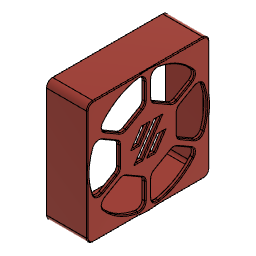
[a]_60mm_fan_blank_insert_x2 (Autodesk Fusion 360 design; units mm, degrees)
Autodesk Fusion 360 part; units mm, degrees
note: some values were not read from the file. Set by a fixed rule: which sketch regions a step uses.
sketch "Master" plane through (0, 0, 0) normal (1, 0, 0) x (0, 1, 0) in component "[a]_60mm_fan_blank_insert_x2"
  line L0 (30, -30) -> (-30, -30)
  line L1 (-30, -30) -> (-30, 30)
  line L2 (-30, 30) -> (30, 30)
  line L3 (30, 30) -> (30, -30)
  line L4 (30, -30) -> (-30, 30) construction
  line L5 (-30, -30) -> (30, 30) construction
  line L6 (-3, 14.4679) -> (-11.0296, 9.8321)
  line L7 (-14.0296, 4.6359) -> (-14.0296, -4.6359)
  line L8 (-11.0296, -9.8321) -> (-3, -14.4679)
  line L9 (3, -14.4679) -> (11.0296, -9.8321)
  line L10 (14.0296, -4.6359) -> (14.0296, 4.6359)
  line L11 (11.0296, 9.8321) -> (3, 14.4679)
  line L12 (-1.5, 25.3537) -> (-1.5, 17.066)
  line L13 (0, 0) -> (0, 50) construction
  line L14 (1.5, 25.3537) -> (1.5, 17.066)
  line L15 (-22.707, 11.3778) -> (-15.5296, 7.234)
  line L16 (-21.207, 13.9759) -> (-14.0296, 9.8321)
  line L17 (-21.207, -13.9759) -> (-14.0296, -9.8321)
  line L18 (-22.707, -11.3778) -> (-15.5296, -7.234)
  line L19 (1.5, -25.3537) -> (1.5, -17.066)
  line L20 (-1.5, -25.3537) -> (-1.5, -17.066)
  line L21 (22.707, -11.3778) -> (15.5296, -7.234)
  line L22 (21.207, -13.9759) -> (14.0296, -9.8321)
  line L23 (21.207, 13.9759) -> (14.0296, 9.8321)
  line L24 (22.707, 11.3778) -> (15.5296, 7.234)
  line L25 (-3.3031, 7.0506) -> (0.0865, 7.0506)
  line L26 (0.0865, 7.0506) -> (-4.5489, -0.001)
  line L27 (-4.5489, -0.001) -> (-7.9375, -0.001)
  line L28 (-7.9375, -0.001) -> (-3.3031, 7.0506)
  line L29 (2.9411, 7.0506) -> (6.3297, 7.0506)
  line L30 (6.3297, 7.0506) -> (-2.9401, -7.0506)
  line L31 (-2.9401, -7.0506) -> (-6.3287, -7.0506)
  line L32 (-6.3287, -7.0506) -> (2.9411, 7.0506)
  line L33 (4.5489, -0.001) -> (7.9375, -0.001)
  line L34 (7.9375, -0.001) -> (3.3031, -7.0506)
  line L35 (3.3031, -7.0506) -> (-0.0855, -7.0506)
  line L36 (-0.0855, -7.0506) -> (4.5489, -0.001)
  arc A0 (22.0029, 18.5049) -> (5.0243, 28.3076) centre (0, 0) ccw
  arc A1 (27.0272, -9.8026) -> (27.0272, 9.8026) centre (0, 0) ccw
  arc A2 (5.0243, -28.3076) -> (22.0029, -18.5049) centre (0, 0) ccw
  arc A3 (-22.0029, -18.5049) -> (-5.0243, -28.3076) centre (0, 0) ccw
  arc A4 (-5.0243, 28.3076) -> (-22.0029, 18.5049) centre (0, 0) ccw
  arc A5 (-27.0272, 9.8026) -> (-27.0272, -9.8026) centre (0, 0) ccw
  arc A6 (21.207, 13.9759) -> (22.0029, 18.5049) centre (19.707, 16.574) ccw
  arc A7 (5.0243, 28.3076) -> (1.5, 25.3537) centre (4.5, 25.3537) ccw
  arc A8 (1.5, 17.066) -> (3, 14.4679) centre (4.5, 17.066) ccw
  arc A9 (11.0296, 9.8321) -> (14.0296, 9.8321) centre (12.5296, 12.4301) ccw
  arc A10 (-1.5, 25.3537) -> (-5.0243, 28.3076) centre (-4.5, 25.3537) ccw
  arc A11 (-3, 14.4679) -> (-1.5, 17.066) centre (-4.5, 17.066) ccw
  arc A12 (-14.0296, 9.8321) -> (-11.0296, 9.8321) centre (-12.5296, 12.4301) ccw
  arc A13 (-22.0029, 18.5049) -> (-21.207, 13.9759) centre (-19.707, 16.574) ccw
  arc A14 (-14.0296, 4.6359) -> (-15.5296, 7.234) centre (-17.0296, 4.6359) ccw
  arc A15 (-22.707, 11.3778) -> (-27.0272, 9.8026) centre (-24.207, 8.7798) ccw
  arc A16 (-27.0272, -9.8026) -> (-22.707, -11.3778) centre (-24.207, -8.7798) ccw
  arc A17 (-15.5296, -7.234) -> (-14.0296, -4.6359) centre (-17.0296, -4.6359) ccw
  arc A18 (-11.0296, -9.8321) -> (-14.0296, -9.8321) centre (-12.5296, -12.4301) ccw
  arc A19 (-21.207, -13.9759) -> (-22.0029, -18.5049) centre (-19.707, -16.574) ccw
  arc A20 (-5.0243, -28.3076) -> (-1.5, -25.3537) centre (-4.5, -25.3537) ccw
  arc A21 (-1.5, -17.066) -> (-3, -14.4679) centre (-4.5, -17.066) ccw
  arc A22 (3, -14.4679) -> (1.5, -17.066) centre (4.5, -17.066) ccw
  arc A23 (14.0296, -9.8321) -> (11.0296, -9.8321) centre (12.5296, -12.4301) ccw
  arc A24 (22.0029, -18.5049) -> (21.207, -13.9759) centre (19.707, -16.574) ccw
  arc A25 (1.5, -25.3537) -> (5.0243, -28.3076) centre (4.5, -25.3537) ccw
  arc A26 (22.707, -11.3778) -> (27.0272, -9.8026) centre (24.207, -8.7798) ccw
  arc A27 (27.0272, 9.8026) -> (22.707, 11.3778) centre (24.207, 8.7798) ccw
  arc A28 (15.5296, 7.234) -> (14.0296, 4.6359) centre (17.0296, 4.6359) ccw
  arc A29 (14.0296, -4.6359) -> (15.5296, -7.234) centre (17.0296, -4.6359) ccw
  dimension "d2" = 60
  dimension "d3" = 60
  dimension "d4" = 57.5
  dimension "d14" = 1.5
  dimension "d15" = 3
  constraint horizontal L0
  constraint perpendicular L0 L1
  constraint parallel L0 L2
  constraint parallel L1 L3
  constraint coincident L4 L13.start
  constraint coincident L5 L13.start
  constraint coincident L13.start A0.centre
  constraint vertical L13
  constraint vertical L12
  constraint concentric A0 A4
  constraint concentric A1 A4
  constraint concentric A2 A4
  constraint concentric A3 A4
  constraint concentric A4 A5
  constraint tangent L23 A6
  constraint tangent A0 A6
  constraint tangent A0 A7
  constraint tangent L14 A7
  constraint equal A6 A7
  constraint tangent L11 A8
  constraint tangent L14 A8
  constraint equal A6 A8
  constraint tangent L23 A9
  constraint tangent L11 A9
  constraint equal A6 A9
  constraint tangent L12 A10
  constraint tangent A4 A10
  constraint equal A6 A10
  constraint tangent L12 A11
  constraint tangent L6 A11
  constraint equal A6 A11
  constraint tangent L6 A12
  constraint tangent L16 A12
  constraint equal A6 A12
  constraint tangent L16 A13
  constraint tangent A4 A13
  constraint equal A6 A13
  constraint tangent L15 A14
  constraint tangent L7 A14
  constraint equal A6 A14
  constraint tangent L15 A15
  constraint tangent A5 A15
  constraint equal A6 A15
  constraint tangent L18 A16
  constraint tangent A5 A16
  constraint equal A6 A16
  constraint tangent L18 A17
  constraint tangent L7 A17
  constraint equal A6 A17
  constraint tangent L17 A18
  constraint tangent L8 A18
  constraint equal A6 A18
  constraint tangent L17 A19
  constraint tangent A3 A19
  constraint equal A6 A19
  constraint tangent L20 A20
  constraint tangent A3 A20
  constraint equal A6 A20
  constraint tangent L20 A21
  constraint tangent L8 A21
  constraint equal A6 A21
  constraint tangent L19 A22
  constraint tangent L9 A22
  constraint equal A6 A22
  constraint tangent L22 A23
  constraint tangent L9 A23
  constraint equal A6 A23
  constraint tangent L22 A24
  constraint tangent A2 A24
  constraint equal A6 A24
  constraint tangent L19 A25
  constraint tangent A2 A25
  constraint equal A6 A25
  constraint tangent L21 A26
  constraint tangent A1 A26
  constraint equal A6 A26
  constraint tangent L24 A27
  constraint tangent A1 A27
  constraint equal A6 A27
  constraint tangent L24 A28
  constraint tangent L10 A28
  constraint equal A6 A28
  constraint tangent L21 A29
  constraint tangent L10 A29
  constraint equal A6 A29
  measures "d2" distance of L1.end L2.end
  measures "d3" distance of L0.end L1.end
  measures "d4" diameter of A4
  measures "d14" distance of L13 L14
  measures "d15" radius of A6
sketch "Outer Square" plane through (0, 0, 0) normal (1, 0, 0) x (0, 1, 0) in component "[a]_60mm_fan_blank_insert_x2"
  line L0 (-30, 30) -> (30, 30)
  line L1 (-30, -30) -> (-30, 30)
  line L2 (30, -30) -> (-30, -30)
  line L3 (30, 30) -> (30, -30)
extrude "Extrude1" add sketch "Outer Square" against normal blind 20 in component "[a]_60mm_fan_blank_insert_x2"
fillet "Fillet1" radius 3 4 edges at (-10, 30, 30) (-10, -30, 30) (-10, 30, -30) (-10, -30, -30) in component "[a]_60mm_fan_blank_insert_x2"
shell "Shell1" thickness 1.6 removed faces 1 at (-20, -11, -10) in component "[a]_60mm_fan_blank_insert_x2"
extrude "Extrude2" cut sketch "Master" against normal blind 1.6 contours L6 L12 L16 A4 A10 A11 A12 A13 | L7 L15 L18 A5 A14 A15 A16 A17 | L8 L17 L20 A3 A18 A19 A20 A21 | L9 L19 L22 A2 A22 A23 A24 A25 | L10 L21 L24 A1 A26 A27 A28 A29 | L11 L14 L23 A0 A6 A7 A8 A9 | L25 L26 L27 L28 | L29 L30 L31 L32 | L33 L34 L35 L36 in component "[a]_60mm_fan_blank_insert_x2"
chamfer "Chamfer1" distance 0.4 angle 45 68 edges at (0, -14.375, 24.8982) (0, -2.5729, 27.653) (0, -1.5, 21.2099) (0, -1.9019, 15.566) (0, -7.0148, 12.15) (0, -12.5296, 9.4301) (0, -17.6183, 11.904) (0, -22.6617, 16.0547) (0, -25.2346, 11.5983) (0, -19.1183, 9.3059) (0, -14.4315, 6.1359) (0, -14.0296, 0) (0, -14.4315, -6.1359) (0, -19.1183, -9.3059) (0, -25.2346, -11.5983) (0, -28.75, 0) (0, -17.6183, -11.904) (0, -12.5296, -9.4301) (0, -7.0148, -12.15) (0, -1.9019, -15.566) (0, -1.5, -21.2099) (0, -2.5729, -27.653) (0, -14.375, -24.8982) (0, -22.6617, -16.0547) (0, 1.5, -21.2099) (0, 1.9019, -15.566) (0, 7.0148, -12.15) (0, 12.5296, -9.4301) (0, 17.6183, -11.904) (0, 22.6617, -16.0547) (0, 14.375, -24.8982) (0, 2.5729, -27.653) (0, 19.1183, -9.3059) (0, 14.4315, -6.1359) (0, 14.0296, 0) (0, 14.4315, 6.1359) (0, 19.1183, 9.3059) (0, 25.2346, 11.5983) (0, 28.75, 0) (0, 25.2346, -11.5983) (0, 12.5296, 9.4301) (0, 7.0148, 12.15) (0, 1.9019, 15.566) (0, 1.5, 21.2099) (0, 2.5729, 27.653) (0, 14.375, 24.8982) (0, 22.6617, 16.0547) (0, 17.6183, 11.904) (0, 30, 0) (0, 29.1213, -29.1213) (0, 0, -30) (0, -29.1213, -29.1213) (0, -30, 0) (0, -29.1213, 29.1213) (0, 0, 30) (0, 29.1213, 29.1213) (0, -5.6203, 3.5248) (0, -6.2432, -0.001) (0, -2.2312, 3.5248) (0, -1.6083, 7.0506) (0, -1.6938, 0) (0, -4.6344, -7.0506) (0, 1.6948, 0) (0, 4.6354, 7.0506) (0, 2.2317, -3.5258) (0, 6.2432, -0.001) (0, 5.6203, -3.5258) (0, 1.6088, -7.0506) in component "[a]_60mm_fan_blank_insert_x2"
sketch "Sketch3" plane through (0, 0, 0) normal (1, 0, 0) x (0, 1, 0) in component "[a]_60mm_fan_blank_insert_x2"
  line L0 (7.0713, 7.4506) -> (-2.7244, -7.4506)
  line L1 (-2.7244, -7.4506) -> (-7.0703, -7.4506)
  line L2 (-7.0703, -7.4506) -> (2.7254, 7.4506)
  line L3 (2.7254, 7.4506) -> (7.0713, 7.4506)
  arc A0 (29.6, 27) -> (27, 29.6) centre (27, 27) ccw
  arc A1 (-27, 29.6) -> (-29.6, 27) centre (-27, 27) ccw
  arc A2 (-29.6, -27) -> (-27, -29.6) centre (-27, -27) ccw
  arc A3 (27, -29.6) -> (29.6, -27) centre (27, -27) ccw
  line L4 (22.507, -11.7242) -> (15.3296, -7.5804)
  arc A4 (13.6296, -4.6359) -> (15.3296, -7.5804) centre (17.0296, -4.6359) ccw
  line L5 (13.6296, -4.6359) -> (13.6296, 4.6359)
  arc A5 (15.3296, 7.5804) -> (13.6296, 4.6359) centre (17.0296, 4.6359) ccw
  line L6 (15.3296, 7.5804) -> (22.507, 11.7242)
  arc A6 (27.4033, 9.939) -> (22.507, 11.7242) centre (24.207, 8.7798) ccw
  arc A7 (27.4033, -9.939) -> (27.4033, 9.939) centre (0, 0) ccw
  arc A8 (22.507, -11.7242) -> (27.4033, -9.939) centre (24.207, -8.7798) ccw
  line L7 (-21.407, -13.6295) -> (-14.2296, -9.4856)
  arc A9 (-10.8296, -9.4856) -> (-14.2296, -9.4856) centre (-12.5296, -12.4301) ccw
  line L8 (-10.8296, -9.4856) -> (-2.8, -14.1215)
  arc A10 (-1.1, -17.066) -> (-2.8, -14.1215) centre (-4.5, -17.066) ccw
  line L9 (-1.1, -17.066) -> (-1.1, -25.3537)
  arc A11 (-5.0942, -28.7014) -> (-1.1, -25.3537) centre (-4.5, -25.3537) ccw
  arc A12 (-22.3091, -18.7624) -> (-5.0942, -28.7014) centre (0, 0) ccw
  arc A13 (-21.407, -13.6295) -> (-22.3091, -18.7624) centre (-19.707, -16.574) ccw
  arc A14 (-5.0942, 28.7014) -> (-22.3091, 18.7624) centre (0, 0) ccw
  arc A15 (-1.1, 25.3537) -> (-5.0942, 28.7014) centre (-4.5, 25.3537) ccw
  line L10 (-1.1, 25.3537) -> (-1.1, 17.066)
  arc A16 (-2.8, 14.1215) -> (-1.1, 17.066) centre (-4.5, 17.066) ccw
  line L11 (-2.8, 14.1215) -> (-10.8296, 9.4856)
  arc A17 (-14.2296, 9.4856) -> (-10.8296, 9.4856) centre (-12.5296, 12.4301) ccw
  line L12 (-14.2296, 9.4856) -> (-21.407, 13.6295)
  arc A18 (-22.3091, 18.7624) -> (-21.407, 13.6295) centre (-19.707, 16.574) ccw
  arc A19 (-22.507, 11.7242) -> (-27.4033, 9.939) centre (-24.207, 8.7798) ccw
  line L13 (-22.507, 11.7242) -> (-15.3296, 7.5804)
  arc A20 (-13.6296, 4.6359) -> (-15.3296, 7.5804) centre (-17.0296, 4.6359) ccw
  line L14 (-13.6296, 4.6359) -> (-13.6296, -4.6359)
  arc A21 (-15.3296, -7.5804) -> (-13.6296, -4.6359) centre (-17.0296, -4.6359) ccw
  line L15 (-15.3296, -7.5804) -> (-22.507, -11.7242)
  arc A22 (-27.4033, -9.939) -> (-22.507, -11.7242) centre (-24.207, -8.7798) ccw
  arc A23 (-27.4033, 9.939) -> (-27.4033, -9.939) centre (0, 0) ccw
  line L16 (1.1, -25.3537) -> (1.1, -17.066)
  arc A24 (2.8, -14.1215) -> (1.1, -17.066) centre (4.5, -17.066) ccw
  line L17 (2.8, -14.1215) -> (10.8296, -9.4856)
  arc A25 (14.2296, -9.4856) -> (10.8296, -9.4856) centre (12.5296, -12.4301) ccw
  line L18 (14.2296, -9.4856) -> (21.407, -13.6295)
  arc A26 (22.3091, -18.7624) -> (21.407, -13.6295) centre (19.707, -16.574) ccw
  arc A27 (5.0942, -28.7014) -> (22.3091, -18.7624) centre (0, 0) ccw
  arc A28 (1.1, -25.3537) -> (5.0942, -28.7014) centre (4.5, -25.3537) ccw
  arc A29 (10.8296, 9.4856) -> (14.2296, 9.4856) centre (12.5296, 12.4301) ccw
  line L19 (10.8296, 9.4856) -> (2.8, 14.1215)
  arc A30 (1.1, 17.066) -> (2.8, 14.1215) centre (4.5, 17.066) ccw
  line L20 (1.1, 17.066) -> (1.1, 25.3537)
  arc A31 (5.0942, 28.7014) -> (1.1, 25.3537) centre (4.5, 25.3537) ccw
  arc A32 (22.3091, 18.7624) -> (5.0942, 28.7014) centre (0, 0) ccw
  arc A33 (21.407, 13.6295) -> (22.3091, 18.7624) centre (19.707, 16.574) ccw
  line L21 (21.407, 13.6295) -> (14.2296, 9.4856)
  line L22 (0.8281, 7.4506) -> (-4.3332, -0.401)
  line L23 (-4.3332, -0.401) -> (-8.679, -0.401)
  line L24 (-8.679, -0.401) -> (-3.5189, 7.4506)
  line L25 (-3.5189, 7.4506) -> (0.8281, 7.4506)
  line L26 (8.6792, 0.399) -> (3.5188, -7.4506)
  line L27 (3.5188, -7.4506) -> (-0.8271, -7.4506)
  line L28 (-0.8271, -7.4506) -> (4.3332, 0.399)
  line L29 (4.3332, 0.399) -> (8.6792, 0.399)
  circle A34 centre (0, 0) radius 30
  circle A35 centre (0, 0) radius 29.2
  dimension "d19" = 60
  dimension "d20" = 58.4
  constraint coincident A7.centre A12.centre
  constraint concentric A7 A35
  measures "d19" diameter of A34
  measures "d20" diameter of A35
extrude "Extrude3" add sketch "Sketch3" against normal blind 1.6 contours A34 in component "[a]_60mm_fan_blank_insert_x2"
component "[a]_60mm_fan_blank_insert_x2" placed x (1, 0, 0) y (0, 1, 0) z (0, 0, 1) at (0, 0, 0)
equation "fan_size = 60 mm"
equation "d2 = fan_size"
equation "d3 = fan_size"
equation "d4 = fan_size - 2.5 mm"
equation "d19 = fan_size"
equation "d20 = fan_size - 1.6 mm"
